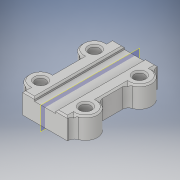
# Autodesk Inventor part: belt_tension_clamp
Saved by Autodesk Inventor 2019 (Build 230136000, 136)
## iProperties
Created: 2020-01-19
Part Number: belt_tension_clamp
Material: Generisch
Document SubType Name: Modeling
Designer: marc
Density: 1 g/cm^3
Appearance: Vorgabe
Author: marc
## iProperties of the stored document belt_tension_clamp_3D-Druck.ipt
Created: 2020-01-19
Part Number: belt_tension_clamp_3D-Druck
Material: Generisch
Document SubType Name: Modeling
Designer: marc
Density: 1 g/cm^3
Appearance: Vorgabe
Author: marc
Autodesk Inventor part; units mm, degrees
ref_plane "YZ Plane" through (0, 0, 0) normal (1, 0, 0) x (0, 1, 0)
ref_plane "XZ Plane" through (0, 0, 0) normal (0, 1, 0) x (-1, 0, 0)
ref_plane "XY Plane" through (0, 0, 0) normal (0, 0, 1) x (1, 0, 0)
sketch "Skizze4" plane through (0, 0, 0) normal (0, 1, 0) x (-1, 0, 0)
  line L0 (0, 0) -> (15, 0)
  line L1 (15, 0) -> (15, 30)
  line L2 (15, 30) -> (0, 30)
  line L3 (0, 30) -> (0, 0)
  dimension "d10" = 15
  dimension "d11" = 30
  constraints: 8 end point, 2 parallel, 1 horizontal, 1 perpendicular
  measures "d10" distance of L2.end L1.end
  measures "d11" distance of L1.end L0.end
extrude "Extrusion3" add sketch "Skizze4" along normal blind 7
sketch "Skizze5" plane through (0, 0, 0) normal (0, 0, -1) x (-1, 0, 0)
  line L0 (11, 7) -> (4, 7)
  line L1 (4, 7) -> (4, 5.95)
  line L2 (4, 5.95) -> (11, 5.95)
  line L3 (11, 5.95) -> (11, 7)
  line L4 (0, 7) -> (15, 7) projected
  line L5 (15, 0) -> (15, 7) projected
  point P0 (0, 0)
  dimension "d14" = 1.05
  dimension "d15" = 7
  dimension "d16" = 4
  constraints: 8 end point, 2 parallel, 1 horizontal, 1 perpendicular, 1 point on line
  measures "d14" distance of L2.end L0.start
  measures "d15" distance of L1.end L2.end
  measures "d16" distance between parallel lines of L5 L3
extrude "Extrusion4" cut sketch "Skizze5" against normal up to next
sketch "Skizze6" plane through (0, 0, 0) normal (0, -1, 0) x (1, 0, 0)
  line L0 (0, 30) -> (0, 0) projected
  circle A0 centre (0, 6) radius 4
  circle A1 centre (0, 24) radius 4
  dimension "d19" = 8
  dimension "d20" = 8
  dimension "d21" = 6
  dimension "d22" = 6
  constraints: 2 centre point, 2 point on line
  measures "d19" diameter of A0
  measures "d20" diameter of A1
  measures "d21" distance of L0.end A0.centre
  measures "d22" distance of L0.start A1.centre
extrude "Extrusion5" add sketch "Skizze6" against normal blind 7
sketch "Skizze7" plane through (0, 0, 0) normal (0, -1, 0) x (1, 0, 0)
  line L0 (-15, 30) -> (0, 30) projected
  line L1 (0, 2) -> (0, 0) projected
  line L2 (0, 30) -> (0, 28) projected
  point P0 (0, 6)
  point P1 (0, 24)
  dimension "d25" = 6
  dimension "d26" = 6
  constraints: 2 point on line
  measures "d25" distance of L1.end point (0, 6)
  measures "d26" distance from line of L0 point (0, 24)
hole "Bohrung1" at (0, 0, 6) at (0, 0, 24) direction (0, 1, 0) diameter 3.3 end through all both
ref_plane "Arbeitsebene1" through (-7.5, 0, 0) normal (-1, 0, 0) x (0, 0, 1)
mirror "Spiegeln1" about plane through (-7.5, 0, 0) normal (-1, 0, 0) of "Extrusion5"
sketch "Skizze8" plane through (0, 0, 0) normal (0, -1, 0) x (1, 0, 0)
  line L0 (-18.1754, 6) -> (-16.5877, 8.75)
  line L1 (-16.5877, 8.75) -> (-13.4123, 8.75)
  line L2 (-13.4123, 8.75) -> (-11.8246, 6)
  line L3 (-11.8246, 6) -> (-13.4123, 3.25)
  line L4 (-13.4123, 3.25) -> (-16.5877, 3.25)
  line L5 (-16.5877, 3.25) -> (-18.1754, 6)
  line L6 (-18.1754, 24) -> (-16.5877, 26.75)
  line L7 (-16.5877, 26.75) -> (-13.4123, 26.75)
  line L8 (-13.4123, 26.75) -> (-11.8246, 24)
  line L9 (-11.8246, 24) -> (-13.4123, 21.25)
  line L10 (-13.4123, 21.25) -> (-16.5877, 21.25)
  line L11 (-16.5877, 21.25) -> (-18.1754, 24)
  line L12 (-15, 10) -> (-15, 20) projected
  line L13 (0, 0) -> (-15, 0) projected
  line L14 (-15, 30) -> (0, 30) projected
  point P0 (-15, 6)
  point P1 (-15, 24)
  dimension "d34" = 5.5
  dimension "d35" = 5.5
  dimension "d36" = 6
  dimension "d37" = 6
  constraints: 24 end point, 2 point on line, 1 horizontal, 1 parallel, 26 other
  measures "d34" distance between parallel lines of L4 L1
  measures "d35" distance between parallel lines of L7 L10
  measures "d36" distance from line of L13 point (-15, 6)
  measures "d37" distance from line of L14 point (-15, 24)
extrude "Extrusion6" cut sketch "Skizze8" against normal blind 3
mirror "Spiegeln2" about plane through (-7.5, 0, 0) normal (-1, 0, 0) of "Bohrung1"
chamfer "Fase1" distance 0.5 angle 45 20 edges at (-11, 7, 15) (-4, 7, 15) (0, 7, 15) (0, 7, 29) (4, 7, 24) (4, 7, 6) (0, 7, 1) (-2, 7, 0) (-2, 7, 30) (-13, 7, 30) (-19, 7, 24) (-15, 7, 29) (-15, 7, 15) (-19, 7, 6) (-15, 7, 1) (-13, 7, 0) (-15, 7, 7.65) (-15, 7, 25.65) (0, 7, 25.65) (0, 7, 7.65)
fillet "Rundung1" radius 2 8 edges at (-15, 3.25, 2) (-15, 3.25, 20) (-15, 3.25, 10) (-15, 3.25, 28) (0, 3.25, 2) (0, 3.25, 20) (0, 3.25, 10) (0, 3.25, 28)
equation "\"d22\" = d21"
equation "\"d35\" = d34"
